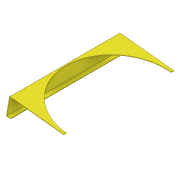
# Autodesk Inventor part: CarouselRamp
Saved by Autodesk Inventor 2018 (Build 220112000, 112)
## iProperties
Created: 2020-02-05
Part Number: CarouselRamp
Material: Polycarbonate, Smoke
Document SubType Name: Modeling
Designer: Myers
Mass: 423.962 g
Surface Area: 2374.43 cm^2
Volume: 353.302 cm^3
Density: 1.2 g/cm^3
Appearance: Canary
Author: Myers
Autodesk Inventor part; units mm, degrees
ref_plane "YZ Plane" through (0, 0, 0) normal (1, 0, 0) x (0, 1, 0)
ref_plane "XZ Plane" through (0, 0, 0) normal (0, 1, 0) x (-1, 0, 0)
ref_plane "XY Plane" through (0, 0, 0) normal (0, 0, 1) x (1, 0, 0)
sketch "Sketch1" plane through (0, 0, 0) normal (0, 0, 1) x (1, 0, 0)
  line L0 (3.739, 2.921) -> (19.8226, 94.1354)
  line L1 (304.8, 66.421) -> (304.8011, 69.342)
  line L2 (304.8011, 69.342) -> (20.634, 99.9646)
  line L3 (17.1671, 97.3593) -> (0, 0)
  line L4 (0, 0) -> (25.4, 0)
  line L5 (25.4, 0) -> (25.4, 2.921)
  line L6 (25.4, 2.921) -> (3.739, 2.921)
  line L7 (23.2893, 96.7408) -> (304.8, 66.421)
  arc A0 (20.634, 99.9646) -> (17.1671, 97.3593) centre (20.2938, 96.8079) ccw
  arc A1 (23.2893, 96.7408) -> (19.8226, 94.1354) centre (22.9493, 93.584) ccw
  point P0 (20.338, 97.0586)
  point P1 (17.6825, 100.2827)
  dimension "d4" = 101.6
  dimension "d12" = 3.175
  dimension "d13" = 25.4
  dimension "d14" = 2.921
  dimension "d15" = 304.8
  dimension "d17" = 80
  dimension "d19" = 2.921
  dimension "d21" = 63.5
  dimension "d24" = 2.921
  dimension "d25" = 93.849
  dimension "d26" = 3.175
  constraints: 16 end point, 4 point on circle, 4 point on line, 4 tangent, 2 centre point, 1 equal length, 1 equal radius, 1 horizontal, 1 parallel, 1 perpendicular, 1 vertical
  measures "d4" distance from line of L2 L3.end
  measures "d12" distance between parallel lines of L0 L3
  measures "d13" distance of L3.end L4.end
  measures "d14" distance of L4.end L5.end
  measures "d15" horizontal distance of L1.start L3.end
  measures "d17" angle of L6 L0
  measures "d19" distance of L1.start L1.end
  measures "d21" distance from line of L6 L1.start
  measures "d24" distance from line of point (20.338, 97.059) L2
  measures "d25" angle of L3 L2
  measures "d26" radius of A0
extrude "Extrusion1" add sketch "Sketch1" along normal mid plane 584.2
sketch "Sketch2" plane through (0, 0, 0) normal (0, 1, 0) x (-1, 0, 0)
  circle A0 centre (-304.8, 0) radius 279.4
  line L0 (0, -292.1) -> (0, 292.1) projected
  point P0 (0, 0)
  point P1 (0, 0)
  dimension "d8" = 558.8
  dimension "d9" = 304.8
  constraints: 1 centre point, 1 horizontal alignment, 1 midpoint
  measures "d8" diameter of A0
  measures "d9" distance from line of L0 A0.centre
extrude "Extrusion2" cut sketch "Sketch2" along normal through all
body "Solid1"
